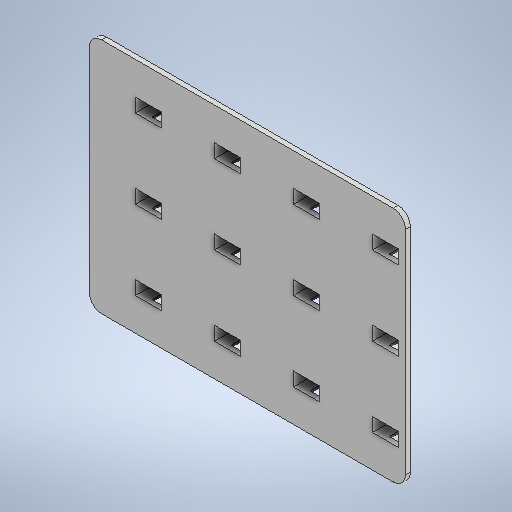
# Autodesk Inventor part: STX2-Plus
Saved by Autodesk Inventor 2025.1 (Build 291241000, 241)
## iProperties
Created: 2023-09-28
Part Number: STX2-Plus
Material: Generic
Document SubType Name: Modeling
Designer: sedm7132
Density: 1 g/cm^3
Appearance: Default
Author: sedm7132
Autodesk Inventor part; units mm, degrees
ref_plane "YZ Plane" through (0, 0, 0) normal (1, 0, 0) x (0, 1, 0)
ref_plane "XZ Plane" through (0, 0, 0) normal (0, 1, 0) x (-1, 0, 0)
ref_plane "XY Plane" through (0, 0, 0) normal (0, 0, 1) x (1, 0, 0)
sketch "Sketch1" plane through (0, 0, 0) normal (0, 0, 1) x (1, 0, 0)
  circle A0 centre (0, 0) radius 6.4
  dimension "d0" = 12.8
  constraints: 1 centre point, 1 coincident
  measures "d0" diameter of A0
extrude "Extrusion1" add sketch "Sketch1" along normal blind 4
sketch "Sketch2" plane through (0, 0, 4) normal (0, 0, 1) x (1, 0, 0)
  line L0 (-12.85, -12.85) -> (12.85, -12.85)
  line L1 (12.85, -12.85) -> (12.85, 12.85)
  line L2 (12.85, 12.85) -> (-12.85, 12.85)
  line L3 (-12.85, 12.85) -> (-12.85, -12.85)
  line L4 (-12.85, -12.85) -> (12.85, 12.85) construction
  line L5 (12.85, -12.85) -> (-12.85, 12.85) construction
  point P0 (0, 0)
  dimension "d3" = 25.7
  dimension "d4" = 25.7
  constraints: 12 end point, 2 midpoint, 2 parallel, 1 horizontal, 1 perpendicular
  measures "d3" distance of L2.end L1.end
  measures "d4" distance of L1.end L0.end
extrude "Extrusion2" add sketch "Sketch2" along normal blind 1.6
sketch "Sketch3" plane through (0, 0, 5.6) normal (0, 0, 1) x (1, 0, 0)
  circle A0 centre (0, 0) radius 6.4 construction
  line L0 (6.35, 0) -> (2.45, 0) construction
  line L1 (6.35, 0) -> (10.45, 0) construction
  line L2 (10.55, -2.25) -> (2.15, -2.25)
  line L3 (2.15, -2.25) -> (2.15, 2.25)
  line L4 (2.15, 2.25) -> (10.55, 2.25)
  line L5 (10.55, 2.25) -> (10.55, -2.25)
  line L6 (10.55, -2.25) -> (2.15, 2.25) construction
  line L7 (2.15, -2.25) -> (10.55, 2.25) construction
  dimension "d12" = 8.4
  dimension "d13" = 4.5
  constraints: 16 end point, 3 horizontal, 2 midpoint, 2 parallel, 1 horizontal alignment, 1 perpendicular, 2 other
  measures "d12" distance of L3.end L4.end
  measures "d13" distance of L4.end L2.start
extrude "Extrusion3" cut sketch "Sketch3" against normal up to surface (5.6 mm away)
pattern_linear "Rectangular Pattern1" count 3 spacing 25.7 along (0, 1, 0) count 4 spacing 25.7 along (1, 0, 0)
fillet "Fillet1" radius 4 4 edges at (-12.85, -12.85, 4.8) (89.95, -12.85, 4.8) (89.95, 64.25, 4.8) (-12.85, 64.25, 4.8)
body "Solid1"
